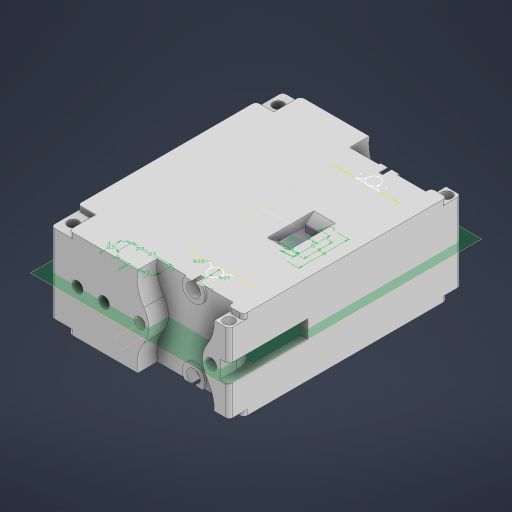
# Autodesk Inventor part: NEW_BODY
Saved by Autodesk Inventor 2024.2 (Build 282272000, 272)
## iProperties
Created: 2024-03-12
Part Number: NEW_BODY
Material: Generic
Document SubType Name: Modeling
Designer: jerem
Density: 1 g/cm^3
Appearance: Default
Author: jerem
## iProperties of the stored document NEW_BODY_3DPrint.ipt
Created: 2024-03-13
Part Number: NEW_BODY_3DPrint
Material: Generic
Document SubType Name: Modeling
Designer: jerem
Density: 1 g/cm^3
Appearance: Default
Author: jerem
Autodesk Inventor part; units mm, degrees
ref_plane "YZ Plane" through (0, 0, 0) normal (1, 0, 0) x (0, 1, 0)
ref_plane "XZ Plane" through (0, 0, 0) normal (0, 1, 0) x (-1, 0, 0)
ref_plane "XY Plane" through (0, 0, 0) normal (0, 0, 1) x (1, 0, 0)
sketch "Sketch1" plane through (0, 0, 0) normal (0, 1, 0) x (-1, 0, 0)
  line L0 (-50, -65) -> (50, -65)
  line L1 (50, -65) -> (50, 65)
  line L2 (50, 65) -> (-50, 65)
  line L3 (-50, 65) -> (-50, -65)
  line L4 (-50, -65) -> (50, 65) construction
  line L5 (50, -65) -> (-50, 65) construction
  point P0 (0, 0)
  dimension "d0" = 130
  dimension "d1" = 100
  constraints: 12 end point, 2 midpoint, 2 parallel, 1 horizontal, 1 perpendicular
  measures "d0" distance of L0.end L1.end
  measures "d1" distance of L1.end L2.end
extrude "Extrusion1" add sketch "Sketch1" along normal blind 50
sketch "Sketch2" plane through (-50, 0, 65) normal (0, 0, 1) x (1, 0, 0)
  line L0 (0, 50) -> (100, 50) projected
  line L1 (100, 50) -> (50, 50)
  line L2 (50, 50) -> (50, 0)
  line L3 (50, 0) -> (100, 0)
  line L4 (100, 0) -> (100, 50)
  constraints: 8 end point, 2 parallel, 1 horizontal, 1 perpendicular
extrude "Extrusion2" cut sketch "Sketch2" against normal blind 15
sketch "Sketch3" plane through (-50, 0, 50) normal (0, 0, 1) x (1, 0, 0)
  circle A0 centre (70, 46.3) radius 3.7
  line L0 (100, 50) -> (100, 0) projected
  line L1 (50, 50) -> (100, 50) projected
  line L2 (50, 0) -> (50, 50) projected
  line L3 (50, 25) -> (100, 25) construction
  circle A1 centre (70, 3.7) radius 3.7
  dimension "d8" = 7.4
  dimension "d95" = 20
  constraints: 2 centre point, 2 end point, 2 midpoint, 1 symmetric about line, 1 tangent, 1 other
  measures "d8" diameter of A0
  measures "d95" distance from line of L2 A0.centre
sketch "Sketch4" plane through (-50, 0, 50) normal (0, 0, 1) x (1, 0, 0)
  circle A0 centre (70, 46.3) radius 3.7 projected
  circle A1 centre (70, 3.7) radius 3.7 projected
  arc A2 (66.7875, 50) -> (73.2125, 50) centre (70, 46.3) ccw
  arc A3 (73.2125, 0) -> (66.7875, 0) centre (70, 3.7) ccw
  line L0 (73.2125, 50) -> (66.7875, 50)
  line L1 (50, 50) -> (100, 50) projected
  line L2 (73.2125, 0) -> (66.7875, 0)
  point P0 (50, 0)
  point P1 (70, 50)
  dimension "d11" = 1.2
  dimension "d12" = 1.2
  dimension "d13" = 6.4249
  dimension "d14" = 6.4249
  constraints: 4 end point, 4 point on circle, 2 centre point, 2 coincident, 1 parallel, 1 point on line, 1 vertical alignment
  measures "d12" radial gap between concentric circles of A1 A3
  measures "d13" distance of L0.start L0.end
  measures "d14" distance of L2.start L2.end
ref_plane "Work Plane1" through (50, 0, 0) normal (0, 0, -1) x (-1, 0, 0)
mirror "Mirror1" about plane through (50, 0, 0) normal (0, 0, -1) of "Extrusion2"
sketch "Sketch5" plane through (0, 0, 0) normal (0, -1, 0) x (1, 0, 0)
  line L0 (-46, -47.5) -> (-4, -47.5)
  line L1 (-4, -47.5) -> (-4, 47.5)
  line L2 (-4, 47.5) -> (-46, 47.5)
  line L3 (-46, 47.5) -> (-46, -47.5)
  line L4 (-46, -47.5) -> (-4, 47.5) construction
  line L5 (-4, -47.5) -> (-46, 47.5) construction
  line L6 (-50, -65) -> (-50, 65) projected
  line L7 (50, 50) -> (50, -50) projected
  line L8 (50, 0) -> (-50, 0) construction
  point P0 (0, 0)
  point P1 (-25, 0)
  dimension "d18" = 4
  dimension "d19" = 42
  dimension "d20" = 95
  constraints: 14 end point, 4 midpoint, 2 parallel, 1 horizontal, 1 perpendicular, 1 point on line
  measures "d18" distance between parallel lines of L6 L3
  measures "d19" distance of L1.end L2.end
  measures "d20" distance of L0.end L1.end
extrude "Extrusion5" cut sketch "Sketch5" against normal blind 30
sketch "Sketch6" plane through (0, 30, 0) normal (0, -1, 0) x (1, 0, 0)
  circle A0 centre (-7.75, -43.75) radius 1.7
  circle A1 centre (-42.25, -43.75) radius 1.7
  circle A2 centre (-42.25, 10.65) radius 1.7
  line L0 (-4, 47.5) -> (-4, -47.5) projected
  line L1 (-46, -47.5) -> (-46, 47.5) projected
  circle A3 centre (-42.25, 10.65) radius 3.75
  circle A4 centre (-42.25, -43.75) radius 3.75
  circle A5 centre (-7.75, -43.75) radius 3.75
  line L2 (-7.75, -43.75) -> (-4, -43.75)
  line L3 (-42.25, -43.75) -> (-46, -43.75)
  line L4 (-4, -47.5) -> (-46, -47.5) projected
  arc A6 (-14.4582, -47.5) -> (-11.4768, -44.1667) centre (-14.4582, -44.5) ccw
  arc A7 (-7.3333, -40.0232) -> (-4, -37.0418) centre (-7, -37.0418) ccw
  arc A8 (-46, -37.0418) -> (-42.6667, -40.0232) centre (-43, -37.0418) ccw
  arc A9 (-38.5232, -44.1667) -> (-35.5418, -47.5) centre (-35.5418, -44.5) ccw
  arc A10 (-42.6667, 6.9232) -> (-46, 3.9418) centre (-43, 3.9418) ccw
  arc A11 (-46, 17.3582) -> (-42.6667, 14.3768) centre (-43, 17.3582) ccw
  point P0 (0, 0)
  point P1 (-42.25, -47.5)
  point P2 (-7.75, -47.5)
  point P3 (-46, 10.65)
  dimension "d23" = 3.4
  dimension "d24" = 3.4
  dimension "d25" = 3.4
  dimension "d26" = 34.5
  dimension "d28" = 54.4
  dimension "d30" = 34.5
  dimension "d34" = 3
  dimension "d35" = 3
  dimension "d36" = 3
  dimension "d37" = 3
  dimension "d38" = 3
  dimension "d39" = 3
  constraints: 20 point on circle, 17 tangent, 12 centre point, 8 point on line, 4 end point, 3 coincident, 1 collinear
  measures "d23" diameter of A2
  measures "d24" diameter of A0
  measures "d25" diameter of A1
  measures "d26" distance of A1.centre A0.centre
  measures "d28" distance of A2.centre A1.centre
  measures "d30" horizontal distance of A0.centre A2.centre
  measures "d34" radius of A11
  measures "d35" radius of A10
  measures "d36" radius of A8
  measures "d37" radius of A9
  measures "d38" radius of A6
  measures "d39" radius of A7
extrude "Extrusion6" add sketch "Sketch6" along normal blind 8 from surface at 0
sketch "Sketch7" plane through (0, 50, 0) normal (0, 1, 0) x (1, 0, 0)
  line L0 (-46, 47.5) -> (-46, -47.5) projected
  line L1 (-46, -47.5) -> (-4, -47.5) projected
  line L2 (-4, -47.5) -> (-4, 47.5) projected
  line L3 (-4, 47.5) -> (-46, 47.5) projected
  line L4 (3, 41) -> (40, 41)
  line L5 (40, 41) -> (40, -41)
  line L6 (40, -41) -> (3, -41)
  line L7 (3, -41) -> (3, 41)
  line L8 (3, 41) -> (40, -41) construction
  line L9 (40, 41) -> (3, -41) construction
  line L10 (-46, 0) -> (-4, 0) construction
  line L11 (-4, -47.5) -> (-4, 47.5) construction
  line L12 (-50, 65) -> (-50, -65) projected
  line L13 (50, -50) -> (50, 50) projected
  point P0 (0, 0)
  point P1 (21.5, 0)
  point P2 (-4, 37.0418)
  dimension "d49" = 37
  dimension "d50" = 82
  dimension "d75" = 10
  constraints: 14 end point, 4 midpoint, 2 parallel, 2 perpendicular, 1 horizontal, 1 point on line
  measures "d49" distance of L5.end L6.end
  measures "d50" distance of L4.end L5.end
  measures "d75" distance between parallel lines of L13 L5
extrude "Extrusion7" cut sketch "Sketch7" against normal blind 30 contours L4 L5 L6 L7
sketch "Sketch9" plane through (0, 50, 0) normal (0, 1, 0) x (1, 0, 0)
  circle A0 centre (21.5, -44.5) radius 3.5
  line L0 (40, -41) -> (3, -41) projected
  line L1 (21.5, -44.5) -> (21.5, -41) construction
  line L2 (3, -41) -> (40, -41) construction
  arc A1 (28.5, -41) -> (25, -44.5) centre (28.5, -44.5) ccw
  arc A2 (18, -44.5) -> (14.5, -41) centre (14.5, -44.5) ccw
  line L3 (40, 41) -> (40, -41) construction
  line L4 (40, 0) -> (3, 0) construction
  line L5 (3, -41) -> (3, 41) construction
  circle A3 centre (21.5, 44.5) radius 3.5
  line L6 (21.5, 44.5) -> (21.5, 41) construction
  arc A4 (25, 44.5) -> (28.5, 41) centre (28.5, 44.5) ccw
  arc A5 (14.5, 41) -> (18, 44.5) centre (14.5, 44.5) ccw
  line L7 (28.5, 41) -> (14.5, 41)
  line L8 (3, 41) -> (40, 41) projected
  point P0 (0, 0)
  point P1 (14.5, -41)
  dimension "d60" = 7
  dimension "d62" = 3.5
  dimension "d63" = 3.5
  constraints: 14 point on circle, 10 end point, 9 symmetric about line, 6 centre point, 5 tangent, 4 midpoint, 4 point on line, 2 collinear, 3 other
  measures "d60" diameter of A0
  measures "d62" radius of A1
  measures "d63" radius of A2
sketch "Sketch10" plane through (0, 0, 0) normal (0, -1, 0) x (1, 0, 0)
  line L0 (-46, -47.5) -> (-46, 47.5) construction
  line L1 (-46, 0) -> (0, 0) construction
  line L2 (-4, -47.5) -> (-46, -47.5) projected
  line L3 (-46, -47.5) -> (-4, -47.5) construction
  circle A0 centre (-25, -52.5) radius 5
  arc A1 (-30, -52.5) -> (-35, -47.5) centre (-35, -52.5) ccw
  arc A2 (-15, -47.5) -> (-20, -52.5) centre (-15, -52.5) ccw
  line L4 (-25, -47.5) -> (-25, -52.5) construction
  line L5 (-4, -47.5) -> (-46, -47.5) construction
  line L6 (-4, 47.5) -> (-46, 47.5)
  line L7 (-46, 47.5) -> (-4, 47.5) construction
  circle A3 centre (-25, 52.5) radius 5
  arc A4 (-35, 47.5) -> (-30, 52.5) centre (-35, 52.5) ccw
  arc A5 (-20, 52.5) -> (-15, 47.5) centre (-15, 52.5) ccw
  line L8 (-25, 47.5) -> (-25, 52.5) construction
  line L9 (-14.4582, 47.5) -> (-35.5418, 47.5) construction
  point P0 (-14.4582, -47.5)
  point P1 (-35.5418, -47.5)
  dimension "d66" = 10
  dimension "d67" = 5
  dimension "d68" = 5
  constraints: 14 end point, 12 point on circle, 12 symmetric about line, 6 centre point, 6 point on line, 5 tangent, 2 horizontal, 2 midpoint, 1 perpendicular, 3 other
  measures "d66" diameter of A0
  measures "d67" radius of A2
  measures "d68" radius of A1
extrude "Extrusion10" cut sketch "Sketch10" against normal blind 3
sketch "Sketch11" plane through (0, 3, 0) normal (0, -1, 0) x (1, 0, 0)
  line L0 (-15, 47.5) -> (-35, 47.5) projected
  arc A0 (-20, 52.5) -> (-15, 47.5) centre (-15, 52.5) ccw projected
  arc A1 (-20, 52.5) -> (-30, 52.5) centre (-25, 52.5) ccw projected
  arc A2 (-35, 47.5) -> (-30, 52.5) centre (-35, 52.5) ccw projected
  line L1 (-35, -47.5) -> (-15, -47.5) projected
  arc A3 (-30, -52.5) -> (-35, -47.5) centre (-35, -52.5) ccw projected
  arc A4 (-30, -52.5) -> (-20, -52.5) centre (-25, -52.5) ccw projected
  arc A5 (-15, -47.5) -> (-20, -52.5) centre (-15, -52.5) ccw projected
  circle A6 centre (-25, -52.5) radius 1.5
  circle A7 centre (-25, 52.5) radius 1.5
  point P0 (0, 0)
  dimension "d71" = 3
  dimension "d72" = 3
  constraints: 2 centre point, 2 coincident
  measures "d71" diameter of A6
  measures "d72" diameter of A7
extrude "Extrusion11" cut sketch "Sketch11" against normal blind 5 contours A6 | A7
sketch "Sketch13" plane through (0, 20, 0) normal (0, 1, 0) x (1, 0, 0)
  line L0 (3, -41) -> (3, 41) projected
  line L1 (3, -41) -> (13, -41)
  line L2 (13, -41) -> (13, -21)
  line L3 (13, -21) -> (3, -21)
  line L4 (3, -21) -> (3, -41)
  point P0 (0, 0)
  point P1 (3, -21)
  dimension "d76" = 20
  dimension "d77" = 10
  constraints: 8 end point, 2 parallel, 1 horizontal, 1 perpendicular
  measures "d76" distance of L1.end L2.end
  measures "d77" distance of L2.end L3.end
revolve "Revolution1" cut sketch "Sketch13" angle 225 about axis through (3, 20, 41) along (0, 0, 1)
ref_plane "Work Plane5" through (0, 47, 0) normal (0, 1, 0) x (1, 0, 0)
sketch "Sketch16" plane through (40, 50, -41) normal (-1, 0, 0) x (0, 0, 1)
  line L0 (47.9232, -20) -> (48.917, -28) projected
  line L1 (0, -30) -> (82, -30) projected
  line L2 (82, -30) -> (62, -30)
  line L3 (62, -30) -> (62, -20)
  line L4 (62, -20) -> (82, -20)
  line L5 (82, -20) -> (82, -30)
  point P0 (41, -50)
  dimension "d83" = 20
  dimension "d84" = 10
  constraints: 8 end point, 2 parallel, 1 horizontal, 1 perpendicular
  measures "d83" distance of L3.end L4.end
  measures "d84" distance of L2.end L3.end
extrude "Extrusion13" cut sketch "Sketch16" against normal up to surface (10 mm away)
sketch "Sketch17" plane through (-50, 0, -65) normal (0, 0, -1) x (-1, 0, 0)
  line L0 (0, 0) -> (0, 50) construction
  line L1 (0, 25) -> (-15, 25) construction
  circle A0 centre (-15, 25) radius 3
  line L2 (-15, 25) -> (-29.8, 25) construction
  circle A1 centre (-29.8, 25) radius 3
  point P0 (-50, 0)
  dimension "d87" = 6
  dimension "d88" = 15
  dimension "d145" = 6
  dimension "d146" = 14.8
  constraints: 4 end point, 2 centre point, 2 coincident, 2 horizontal, 1 midpoint
  measures "d87" diameter of A0
  measures "d88" distance of L1.start L1.end
  measures "d145" diameter of A1
  measures "d146" distance of L2.start L2.end
extrude "Extrusion14" cut sketch "Sketch17" against normal blind 10
mirror "Mirror2" about plane through (0, 0, 0) normal (0, 0, 1) of "Extrusion14"
ref_plane "Work Plane3" through (16.7875, 0, -50) normal (0, 0, -1) x (-1, 0, 0)
sketch "Sketch18" plane through (16.7875, 0, -50) normal (0, 0, -1) x (-1, 0, 0)
  circle A0 centre (-3.2125, 46.3) radius 17.5 construction
  circle A1 centre (-3.2125, 3.7) radius 17.5 construction
  line L0 (-33.2125, 50) -> (-33.2125, 0) projected
  line L1 (-33.2125, 0) -> (-33.2125, 50)
  arc A2 (-33.2125, 10) -> (-33.2125, 40) centre (-33.2125, 25) ccw
  line L2 (26.8875, 50) -> (26.8875, 0)
  arc A3 (26.8875, 40) -> (26.8875, 10) centre (26.8875, 25) ccw
  point P0 (16.7875, 0)
  point P1 (-33.2125, 10)
  point P2 (26.8875, 10)
  point P3 (26.8875, 40)
  dimension "d91" = 35
  dimension "d92" = 35
  dimension "d96" = 30
  constraints: 4 centre point, 4 end point, 4 point on circle, 2 point on line, 1 midpoint
  measures "d91" diameter of A0
  measures "d92" diameter of A1
  measures "d96" diameter of A2
extrude "Extrusion15" add sketch "Sketch18" along normal up to surface (15 mm away)
ref_plane "Work Plane4" through (50, 25, -65) normal (0, 0, -1) x (-1, 0, 0)
sketch "Sketch19" plane through (50, 25, -65) normal (0, 0, -1) x (-1, 0, 0)
  arc A0 (0, -15) -> (0, 15) centre (0, 0) ccw construction
  line L0 (0, -15) -> (0, 15) construction
  circle A1 centre (10, 0) radius 3
  circle A2 centre (85, 0) radius 3 construction
  circle A3 centre (50.1, 0) radius 3
  line L1 (15, 0) -> (10, 0)
  arc A4 (50, 11.0901) -> (50, -11.0901) centre (60.1, 0) ccw projected
  line L2 (105.9, -25) -> (-17.65, -25) projected
  point P0 (45.1, 0)
  dimension "d97" = 6
  dimension "d101" = 6
  dimension "d102" = 5
  dimension "d144" = 5
  constraints: 2 centre point, 2 end point, 2 point on circle, 1 coincident, 1 midpoint, 1 parallel, 1 point on line
  measures "d97" diameter of A1
  measures "d101" diameter of A3
  measures "d102" distance of L1.start L1.end
  measures "d144" distance of point (45.1, 0) A3.centre
extrude "Extrusion16" cut sketch "Sketch19" against normal blind 10
sketch "Sketch21" plane through (0, 30, 0) normal (0, -1, 0) x (1, 0, 0)
  line L0 (-34, 47.5) -> (-16, 47.5)
  line L1 (-16, 47.5) -> (-16, 35.3)
  line L2 (-16, 35.3) -> (-34, 35.3)
  line L3 (-34, 35.3) -> (-34, 47.5)
  line L4 (-34, 47.5) -> (-46, 47.5) construction
  line L5 (-46, -47.5) -> (-46, 47.5) construction
  line L6 (-16, 47.5) -> (-4, 47.5) construction
  line L7 (-4, 47.5) -> (-4, -47.5) construction
  line L8 (-15, 47.5) -> (-35, 47.5) construction
  circle A0 centre (-36.25, 41.4) radius 1.5
  circle A1 centre (-13.75, 41.4) radius 1.5
  line L9 (-34, 41.4) -> (-36.25, 41.4)
  line L10 (-16, 41.4) -> (-13.75, 41.4)
  line L11 (-34, 47.5) -> (-38.75, 47.5)
  line L12 (-38.75, 47.5) -> (-38.75, 35.3)
  line L13 (-38.75, 35.3) -> (-11.25, 35.3)
  line L14 (-11.25, 35.3) -> (-11.25, 47.5)
  line L15 (-16, 47.5) -> (-11.25, 47.5)
  point P0 (0, 0)
  dimension "d108" = 18
  dimension "d110" = 0
  dimension "d202" = 3
  dimension "d203" = 22.5
  dimension "d206" = 3
  dimension "d207" = 12.2
  dimension "d208" = 27.5
  constraints: 26 end point, 6 point on line, 4 collinear, 4 perpendicular, 3 horizontal, 2 centre point, 2 midpoint, 2 parallel, 1 vertical
  measures "d108" distance of L0.start L0.end
  measures "d110" distance between parallel lines of L8 L0
  measures "d202" diameter of A0
  measures "d203" distance of L10.end L9.end
  measures "d206" diameter of A1
  measures "d207" distance of L11.end L12.end
  measures "d208" distance of L12.end L13.end
sketch "Sketch25" plane through (0, 50, 0) normal (0, 1, 0) x (1, 0, 0)
  line L0 (0, 65) -> (-50, 65) projected
  line L1 (-50, 65) -> (-40, 65)
  line L2 (-40, 65) -> (-40, 50)
  line L3 (-40, 50) -> (-50, 50)
  line L4 (-50, 50) -> (-50, 65)
  circle A0 centre (-45, 57.5) radius 3
  line L5 (-50, 65) -> (-50, -65) construction
  line L6 (-50, 0) -> (-20.5898, 0) construction
  point P0 (0, 0)
  point P1 (-30.8869, 65)
  dimension "d129" = 15
  dimension "d130" = 10
  dimension "d131" = 7.5
  dimension "d132" = 6
  dimension "d133" = 5
  constraints: 10 end point, 2 horizontal, 2 parallel, 1 centre point, 1 midpoint, 1 perpendicular
  measures "d129" distance of L1.end L2.end
  measures "d130" distance of L2.end L3.end
  measures "d131" distance from line of L3 A0.centre
  measures "d132" diameter of A0
  measures "d133" distance from line of L2 A0.centre
extrude "Extrusion21" cut sketch "Sketch25" against normal blind 3 contours L2 L3 L4 L0 | A0
extrude "Extrusion22" cut sketch "Sketch25" against normal blind 5 from surface at -3 contours A0
mirror "Mirror4" about plane through (0, 0, 0) normal (0, 0, 1) of "Extrusion21", "Extrusion22"
sketch "Sketch26" plane through (-10.1, 25, -65) normal (0, 0, -1) x (0, -1, 0)
  arc A0 (-11.0901, -10.1) -> (11.0901, -10.1) centre (0, 0) ccw projected
  circle A1 centre (0, -10) radius 3 projected
  circle A2 centre (0, -10) radius 3
  line L0 (0, -10) -> (-11.1803, -10) construction
  line L1 (0, -10) -> (11.1803, -10) construction
  line L2 (-22, 39.9) -> (-22, 29.9) projected
  line L3 (-22, 29.9) -> (-25, 29.9) projected
  line L4 (-25, -10.1) -> (-25, 29.9) projected
  line L5 (-25, -10.1) -> (-11.0901, -10.1) projected
  line L6 (11.0901, -10.1) -> (25, -10.1) projected
  line L7 (25, -10.1) -> (25, 39.9) projected
  line L8 (25, 39.9) -> (-22, 39.9) projected
  point P0 (-10.1, -25)
  constraints: 4 end point, 2 collinear, 2 point on circle, 1 centre point, 1 concentric, 1 horizontal, 1 point on line
extrude "Extrusion23" cut sketch "Sketch26" against normal up to surface (10 mm away) contours A1
ref_plane "Work Plane2" through (0, 25, 0) normal (0, -1, 0) x (1, 0, 0)
mirror "Mirror6" about plane through (0, 25, 0) normal (0, -1, 0) of "Extrusion21", "Extrusion22", "Mirror4"
sketch "Sketch27" plane through (-50, 47, -65) normal (-1, 0, 0) x (0, 0, 1)
  circle A0 centre (65, -22) radius 5
  line L0 (0, -44) -> (0, 0) projected
  line L1 (156, -22) -> (-26, -22) projected
  point P0 (65, -47)
  dimension "d140" = 10
  dimension "d141" = 65
  constraints: 1 centre point, 1 midpoint
  measures "d140" diameter of A0
  measures "d141" distance from line of L0 A0.centre
extrude "Extrusion24" cut sketch "Sketch27" against normal blind 5
mirror "Mirror7" about plane through (0, 0, 0) normal (0, 0, 1) of "Extrusion15"
sketch "Sketch28" plane through (50, 0, -50) normal (0, 0, -1) x (-1, 0, 0)
  circle A0 centre (10, 25) radius 3 projected
  line L0 (10, 25) -> (30, 25) construction
  line L1 (30, 25) -> (30, 46) construction
  circle A1 centre (30, 46) radius 3.5
  circle A2 centre (30, 46) radius 6.5
  line L2 (35.1235, 50) -> (24.8765, 50)
  line L3 (35.5, 50) -> (32, 50) projected
  line L4 (0, 50) -> (50, 50) projected
  line L5 (30, 49.5) -> (30, 50)
  line L6 (25, 50) -> (32, 50) projected
  line L7 (29, 50) -> (29, 49.3541)
  line L8 (31, 50) -> (31, 49.3541)
  point P0 (50, 0)
  dimension "d147" = 20
  dimension "d148" = 21
  dimension "d149" = 7
  dimension "d150" = 3
  dimension "d237" = 1
  constraints: 12 end point, 4 point on circle, 3 perpendicular, 3 point on line, 2 centre point, 2 coincident, 2 symmetric about line, 1 collinear, 1 horizontal, 1 line through centre
  measures "d147" distance of L0.start L0.end
  measures "d148" distance of L0.end L1.end
  measures "d149" diameter of A1
  measures "d150" radial gap between concentric circles of A2 A1
  measures "d237" distance between parallel lines of L5 L7
extrude "Extrusion25" add sketch "Sketch28" along normal blind 5 contours A1 L8 L2 A2 L7
mirror "Mirror8" about plane through (0, 25, 0) normal (0, -1, 0) of "Extrusion25"
mirror "Mirror9" about plane through (0, 0, 0) normal (0, 0, 1) of "Extrusion25", "Mirror8"
mirror "Mirror10" about plane through (0, 0, 0) normal (0, 0, 1) of "Extrusion16"
sketch "Sketch29" plane through (-10.1, 25, -65) normal (0, 0, -1) x (-1, 0, 0)
  arc A0 (-10.1, 11.0901) -> (-10.1, -11.0901) centre (0, 0) ccw projected
  line L0 (29.9, -25) -> (-10.1, -25) projected
  arc A1 (-8.7702, -25) -> (-12.3019, -8.5827) centre (-30.1, -21) ccw
  arc A2 (-29.1, -24.3541) -> (-31.1, -24.3541) centre (-30.1, -21) ccw projected
  constraints: 3 point on circle, 1 centre point, 1 concentric, 1 point on line, 1 tangent
sketch "Sketch31" plane through (-50, 0, 50) normal (0, 0, 1) x (1, 0, 0)
  line L0 (100, 50) -> (100, 40) projected
  arc A0 (100, 40) -> (100, 10) centre (100, 25) ccw projected
  line L1 (100, 50) -> (100, 40)
  line L2 (75.1235, 50) -> (100, 50) construction
  arc A1 (87.7115, 33.6019) -> (91.2464, 50) centre (70, 46) ccw
  line L3 (100, 50) -> (91.2464, 50)
  arc A2 (69, 49.3541) -> (71, 49.3541) centre (70, 46) ccw projected
  point P0 (50, 0)
  constraints: 4 end point, 3 point on circle, 1 centre point, 1 collinear, 1 concentric, 1 point on line, 1 tangent, 1 vertical
extrude "Extrusion28" add sketch "Sketch31" along normal up to surface (15 mm away)
mirror "Mirror13" about plane through (0, 25, 0) normal (0, -1, 0) of "Extrusion28"
mirror "Mirror14" about plane through (0, 0, 0) normal (0, 0, 1) of "Extrusion28", "Mirror13"
sketch "Sketch32" plane through (-10.1, 25, -65) normal (0, 0, -1) x (-1, 0, 0)
  arc A0 (-29.1, -24.3541) -> (-31.1, -24.3541) centre (-30.1, -21) ccw construction
  line L0 (-30.1, -21) -> (-30.1, 21.2793) construction
  line L1 (-35.1, 22) -> (-28.1, 22) construction
  arc A1 (-8.7702, -25) -> (-12.3019, -8.5827) centre (-30.1, -21) ccw
  arc A2 (-10.1, 11.0901) -> (-10.1, -11.0901) centre (0, 0) ccw projected
  line L2 (-10.1, -25) -> (-10.1, -11.0901)
  line L3 (-10.1, -11.0901) -> (-10.1, -25) construction
  line L4 (-24.9765, -25) -> (-10.1, -25) projected
  line L5 (-10.1, -25) -> (-8.7702, -25)
  point P0 (-51.3464, -25)
  point P1 (-10.1, -12.5762)
  constraints: 8 end point, 3 point on circle, 2 collinear, 1 centre point, 1 concentric, 1 perpendicular, 1 tangent
extrude "Extrusion29" add sketch "Sketch32" against normal up to surface (15 mm away) contours A1 A2 L2
extrude "Extrusion30" cut sketch "Sketch32" against normal up to surface (15 mm away) contours L5 L2 A1
mirror "Mirror15" about plane through (0, 25, 0) normal (0, -1, 0) of "Extrusion29", "Extrusion30"
mirror "Mirror16" about plane through (0, 0, 0) normal (0, 0, 1) of "Extrusion29", "Extrusion30", "Mirror15"
sketch "Sketch33" plane through (50, 0, -65) normal (1, 0, 0) x (0, 0, -1)
  line L0 (-106, 20) -> (-86, 20) projected
  line L1 (-130, 33.6019) -> (-130, 16.3981) projected
  line L2 (-106, 20) -> (-130, 20)
  line L3 (-130, 20) -> (-130, 30)
  line L4 (-130, 30) -> (-106, 30)
  line L5 (-106, 30) -> (-106, 20)
  point P0 (-65, 0)
  dimension "d167" = 10
  constraints: 8 end point, 2 parallel, 1 horizontal, 1 perpendicular, 1 point on line
  measures "d167" distance of L4.end L0.start
extrude "Extrusion31" cut sketch "Sketch33" against normal blind 5
sketch "Sketch34" plane through (0, 0, 0) normal (0, -1, 0) x (1, 0, 0)
  line L0 (50, 65) -> (50, -65) projected
  line L1 (50, -65) -> (41, -65)
  line L2 (41, -65) -> (41, -57)
  line L3 (41, -57) -> (50, -57)
  line L4 (50, -57) -> (50, -65)
  point P0 (0, 0)
  dimension "d170" = 9
  dimension "d171" = 8
  constraints: 8 end point, 2 parallel, 1 horizontal, 1 perpendicular
  measures "d170" distance of L0.end L1.end
  measures "d171" distance of L1.end L2.end
extrude "Extrusion32" cut sketch "Sketch34" against normal blind 3
sketch "Sketch35" plane through (0, 3, 0) normal (0, -1, 0) x (1, 0, 0)
  circle A0 centre (46, -61) radius 3
  line L0 (50, -57) -> (50, -65) projected
  line L1 (50, -65) -> (41.5965, -65) projected
  point P0 (0, 0)
  point P1 (42, -65)
  dimension "d174" = 6
  dimension "d175" = 4
  dimension "d176" = 4
  constraints: 1 centre point
  measures "d174" diameter of A0
  measures "d175" distance from line of L0 A0.centre
  measures "d176" distance from line of L1 A0.centre
extrude "Extrusion33" cut sketch "Sketch35" against normal blind 11
mirror "Mirror17" about plane through (0, 25, 0) normal (0, -1, 0) of "Extrusion32", "Extrusion33"
mirror "Mirror18" about plane through (0, 0, 0) normal (0, 0, 1) of "Extrusion32", "Extrusion33", "Mirror17"
sketch "Sketch37" plane through (40, 50, -41) normal (-1, 0, 0) x (0, 0, 1)
  line L0 (62, -30) -> (62, -20) projected
  line L1 (62, -20) -> (82, -20) projected
  line L2 (82, 0) -> (82, -20) projected
  line L3 (0, 0) -> (82, 0) projected
  line L4 (0, 0) -> (0, -30) projected
  line L5 (0, -30) -> (62, -30) projected
  line L6 (82, 0) -> (82, -20) projected
  line L7 (82, -5) -> (0, -5)
  point P0 (41, -50)
  point P1 (82, -5)
  dimension "d186" = 5
  constraints: 2 end point, 2 point on line, 1 perpendicular
  measures "d186" distance between parallel lines of L3 L7
extrude "Extrusion34" cut sketch "Sketch37" against normal blind 5 contours L5 L4 L7 L2 L1 L0
fillet "Fillet5" radius 15 1 edges at (45, 25, 41)
fillet "Fillet6" radius 2 17 edges at (50, 25, -65) (50, 11.5, 65) (50, 38.5, 65) (-50, 25, 65) (-50, 25, -65) (-40, 1.5, -65) (-50, 1.5, -50) (-50, 1.5, 50) (-40, 1.5, 65) (41.4739, 1.4939, 57) (41.4739, 48.5061, 57) (-40, 48.5, 65) (-50, 48.5, 50) (41.4739, 48.5061, -57) (-50, 48.5, -50) (-40, 48.5, -65) (41.4739, 1.4939, -57)
fillet "Fillet8" radius 2 4 edges at (50, 48.5, -57) (50, 1.5, -57) (50, 1.5, 57) (50, 48.5, 57)
sketch "Sketch39" plane through (0, 0, 0) normal (0, -1, 0) x (1, 0, 0)
  line L0 (-4, 47.5) -> (-4, -37.0418) projected
  circle A0 centre (-4, 0) radius 7
  point P0 (0, 0)
  point P1 (-4, 21)
  point P2 (-4, 7)
  point P3 (-4, -7)
  dimension "d192" = 14
  constraints: 1 centre point, 1 point on line
  measures "d192" diameter of A0
extrude "Extrusion36" cut sketch "Sketch39" against normal blind 3 contours A0 L0 picked at (-0.6441, -1.6274)
sketch "Sketch40" plane through (20, 46, 55) normal (0, 0, 1) x (1, 0, 0)
  arc A0 (-1, 3.3541) -> (1, 3.3541) centre (0, 0) ccw projected
  circle A1 centre (0, 0) radius 3.85
  point P0 (-20, -46)
  constraints: 1 centre point, 1 coincident
extrude "Extrusion37" cut sketch "Sketch40" against normal up to surface (5 mm away)
mirror "Mirror19" about plane through (0, 25, 0) normal (0, -1, 0) of "Extrusion37"
mirror "Mirror20" about plane through (0, 0, 0) normal (0, 0, 1) of "Extrusion37", "Mirror19"
sketch "Sketch42" plane through (0, 30, 0) normal (0, -1, 0) x (1, 0, 0)
  point P0 (0, 0)
sketch "Sketch43" plane through (0, 30, 0) normal (0, -1, 0) x (1, 0, 0)
  line L0 (-35, -47.5) -> (-15, -47.5)
  line L1 (-15, -47.5) -> (-15, 2.5)
  line L2 (-15, 2.5) -> (-35, 2.5)
  line L3 (-35, 2.5) -> (-35, -47.5)
  line L4 (-35, -47.5) -> (-15, 2.5) construction
  line L5 (-15, -47.5) -> (-35, 2.5) construction
  line L6 (-25, -22.5) -> (-4, -22.5) construction
  line L7 (-4, -7) -> (-4, -47.5) construction
  line L8 (-25, -22.5) -> (-46, -22.5) construction
  line L9 (-46, -47.5) -> (-46, 47.5) construction
  line L10 (-4, -47.5) -> (-15, -47.5) construction
  point P0 (0, 0)
  dimension "d222" = 50
  dimension "d223" = 20
  dimension "d224" = 0
  constraints: 16 end point, 3 point on line, 2 horizontal, 2 midpoint, 2 parallel, 1 collinear, 1 perpendicular
  measures "d222" distance of L0.end L1.end
  measures "d223" distance of L1.end L2.end
  measures "d224" distance between parallel lines of L10 L0
extrude "Extrusion42" cut sketch "Sketch43" against normal blind 7
sketch "Sketch44" plane through (0, 20, 0) normal (0, 1, 0) x (1, 0, 0)
  line L0 (3, -41) -> (-4, -41) projected
  line L1 (45, 41) -> (3, 41)
  line L2 (3, 41) -> (3, -41)
  line L3 (3, -41) -> (45, -41)
  line L4 (45, -41) -> (45, 41)
  point P0 (0, 0)
  constraints: 8 end point, 2 parallel, 1 horizontal, 1 perpendicular
extrude "Extrusion43" add sketch "Sketch44" along normal up to surface (30 mm away)
sketch "Sketch46" plane through (0, 30, 0) normal (0, -1, 0) x (1, 0, 0)
  line L0 (-15, 2.5) -> (-15, -47.5) projected
  line L1 (-14.4582, -47.5) -> (-15, -47.5) projected
  arc A0 (-14.4582, -47.5) -> (-11.4768, -44.1667) centre (-14.4582, -44.5) ccw projected
  arc A1 (-7.3333, -40.0232) -> (-4, -37.0418) centre (-7, -37.0418) ccw projected
  line L2 (-4, 47.5) -> (-4, -37.0418) projected
  line L3 (-46, 47.5) -> (-4, 47.5) projected
  line L4 (-46, 17.3582) -> (-46, 47.5) projected
  arc A2 (-46, 17.3582) -> (-42.6667, 14.3768) centre (-43, 17.3582) ccw projected
  arc A3 (-42.6667, 6.9232) -> (-46, 3.9418) centre (-43, 3.9418) ccw projected
  line L5 (-46, 0) -> (-46, 3.9418) projected
  line L6 (-46, -37.0418) -> (-46, 0) projected
  arc A4 (-46, -37.0418) -> (-42.6667, -40.0232) centre (-43, -37.0418) ccw projected
  arc A5 (-38.5232, -44.1667) -> (-35.5418, -47.5) centre (-35.5418, -44.5) ccw projected
  line L7 (-35, -47.5) -> (-35.5418, -47.5) projected
  line L8 (-35, -47.5) -> (-35, 2.5) projected
  line L9 (-35, 2.5) -> (-15, 2.5) projected
  line L10 (-46, 4) -> (-46, -5) projected
  line L11 (-46, -5) -> (-35, -5)
  line L12 (-42.6667, 14.3768) -> (-32.6667, 14.3768)
  line L13 (-32.6667, 14.3768) -> (-32.6667, 2.5)
  arc A6 (-7.3333, -40.0232) -> (-11.4768, -44.1667) centre (-7.75, -43.75) ccw projected
  arc A7 (-42.6667, 6.9232) -> (-42.6667, 14.3768) centre (-42.25, 10.65) ccw projected
  arc A8 (-38.5232, -44.1667) -> (-42.6667, -40.0232) centre (-42.25, -43.75) ccw projected
  line L14 (-42.6667, 14.3768) -> (-42.6667, 11.2818)
  point P0 (0, 0)
  point P1 (-46, -4.5826)
  point P2 (-46, 4.9552)
  point P3 (-46, -5)
  point P4 (-41.8333, 14.3768)
  dimension "d231" = 10
  constraints: 8 end point, 2 perpendicular, 2 point on line, 1 horizontal, 1 vertical
  measures "d231" distance of L12.start L12.end
extrude "Extrusion45" cut sketch "Sketch46" against normal up to surface (7 mm away)
sketch "Sketch47" plane through (0, 37, 0) normal (0, -1, 0) x (1, 0, 0)
  line L0 (-35.5418, -47.5) -> (-14.4582, -47.5) projected
  arc A0 (-14.4582, -47.5) -> (-11.4768, -44.1667) centre (-14.4582, -44.5) ccw projected
  arc A1 (-7.3333, -40.0232) -> (-11.4768, -44.1667) centre (-7.75, -43.75) ccw projected
  arc A2 (-7.3333, -40.0232) -> (-4, -37.0418) centre (-7, -37.0418) ccw projected
  line L1 (-4, -37.0418) -> (-4, 47.5) projected
  line L2 (-4, 47.5) -> (-46, 47.5) projected
  line L3 (-46, 47.5) -> (-46, 17.3582) projected
  arc A3 (-46, 17.3582) -> (-42.6667, 14.3768) centre (-43, 17.3582) ccw projected
  line L4 (-42.6667, 14.3768) -> (-41.8333, 14.3768) projected
  arc A4 (-42.6667, 6.9232) -> (-41.8333, 14.3768) centre (-42.25, 10.65) ccw projected
  arc A5 (-42.6667, 6.9232) -> (-46, 3.9418) centre (-43, 3.9418) ccw projected
  line L5 (-46, 3.9418) -> (-46, -37.0418) projected
  arc A6 (-46, -37.0418) -> (-42.6667, -40.0232) centre (-43, -37.0418) ccw projected
  arc A7 (-38.5232, -44.1667) -> (-42.6667, -40.0232) centre (-42.25, -43.75) ccw projected
  arc A8 (-38.5232, -44.1667) -> (-35.5418, -47.5) centre (-35.5418, -44.5) ccw projected
  point P0 (0, 0)
extrude "Extrusion46" cut sketch "Sketch47" against normal blind 2
sketch "Sketch51" plane through (-50, 0, 50) normal (0, 0, 1) x (1, 0, 0)
  arc A0 (48.6702, 50) -> (52.2019, 33.5827) centre (70, 46) ccw projected
  arc A1 (52.2019, 16.4173) -> (52.2019, 33.5827) centre (39.9, 25) ccw projected
  arc A2 (52.2019, 16.4173) -> (48.6702, 0) centre (70, 4) ccw projected
  line L0 (64.8765, 0) -> (48.6702, 0) projected
  arc A3 (75.1235, 0) -> (64.8765, 0) centre (70, 4) ccw projected
  line L1 (91.2464, 0) -> (75.1235, 0) projected
  arc A4 (91.2464, 0) -> (87.7115, 16.3981) centre (70, 4) ccw projected
  arc A5 (87.7115, 33.6019) -> (87.7115, 16.3981) centre (100, 25) ccw projected
  arc A6 (87.7115, 33.6019) -> (91.2464, 50) centre (70, 46) ccw projected
  line L2 (75.1235, 50) -> (91.2464, 50) projected
  arc A7 (64.8765, 50) -> (75.1235, 50) centre (70, 46) ccw projected
  line L3 (48.6702, 50) -> (64.8765, 50) projected
  point P0 (50, 0)
extrude "Extrusion47" add sketch "Sketch51" along normal blind 4
sketch "Sketch52" plane through (20, 46, -50) normal (0, 0, -1) x (-1, 0, 0)
  arc A0 (17.7981, -12.4173) -> (21.3298, 4) centre (0, 0) ccw projected
  line L0 (5.1235, 4) -> (21.3298, 4) projected
  arc A1 (-5.1235, 4) -> (5.1235, 4) centre (0, 0) ccw projected
  line L1 (-21.2464, 4) -> (-5.1235, 4) projected
  arc A2 (-21.2464, 4) -> (-17.7115, -12.3981) centre (0, 0) ccw projected
  arc A3 (-17.7115, -29.6019) -> (-17.7115, -12.3981) centre (-30, -21) ccw projected
  arc A4 (-17.7115, -29.6019) -> (-21.2464, -46) centre (0, -42) ccw projected
  line L2 (-5.1235, -46) -> (-21.2464, -46) projected
  arc A5 (5.1235, -46) -> (-5.1235, -46) centre (0, -42) ccw projected
  line L3 (21.3298, -46) -> (5.1235, -46) projected
  arc A6 (21.3298, -46) -> (17.7981, -29.5827) centre (0, -42) ccw projected
  arc A7 (17.7981, -12.4173) -> (17.7981, -29.5827) centre (30.1, -21) ccw projected
  point P0 (20, -46)
extrude "Extrusion48" add sketch "Sketch52" along normal blind 4
sketch "Sketch53" plane through (0, 0, 0) normal (0, -1, 0) x (1, 0, 0)
  line L0 (-46, -47.5) -> (-46, 47.5) projected
  line L1 (-46, 47.5) -> (46, 47.5)
  line L2 (46, 47.5) -> (46, -47.5)
  line L3 (46, -47.5) -> (-46, -47.5)
  line L4 (-46, -47.5) -> (-46, 47.5)
  line L5 (50, 55) -> (50, -55) projected
  point P0 (0, 0)
  dimension "d244" = 4
  constraints: 8 end point, 2 parallel, 1 horizontal, 1 perpendicular
  measures "d244" distance between parallel lines of L5 L2
extrude "Extrusion49" cut sketch "Sketch53" against normal blind 45
sketch "Sketch54" plane through (-46, 0, -47.5) normal (0, 0, 1) x (1, 0, 0)
  circle A0 centre (57.036, 7.7) radius 1.5
  line L0 (92, 5) -> (0, 5)
  line L1 (0, 5) -> (0, 45)
  line L2 (0, 45) -> (92, 45)
  line L3 (92, 45) -> (92, 5)
  line L4 (96, 47) -> (96, 3) projected
  line L5 (-4, 3) -> (-4, 47) projected
  line L6 (60.8765, 0) -> (44.6702, 0) projected
  line L7 (44.6702, 50) -> (8, 50) projected
  line L8 (59.736, 5) -> (59.736, 46.19) construction
  line L9 (-0.264, 5) -> (-0.264, 45) construction
  circle A1 centre (2.436, 7.7) radius 1.5
  line L10 (54.336, 10.4) -> (59.736, 10.4)
  line L11 (59.736, 10.4) -> (59.736, 5)
  line L12 (59.736, 5) -> (54.336, 5)
  line L13 (54.336, 5) -> (54.336, 10.4)
  line L14 (54.336, 10.4) -> (59.736, 5) construction
  line L15 (59.736, 10.4) -> (54.336, 5) construction
  line L16 (5.136, 10.4) -> (-0.264, 10.4)
  line L17 (-0.264, 10.4) -> (-0.264, 5)
  line L18 (-0.264, 5) -> (5.136, 5)
  line L19 (5.136, 5) -> (5.136, 10.4)
  line L20 (5.136, 10.4) -> (-0.264, 5) construction
  line L21 (-0.264, 10.4) -> (5.136, 5) construction
  line L22 (-0.264, 45) -> (5.136, 45) construction
  line L23 (5.136, 45) -> (5.136, 39.6)
  line L24 (5.136, 39.6) -> (-0.264, 39.6)
  line L25 (-0.264, 39.6) -> (-0.264, 45)
  circle A2 centre (2.436, 42.3) radius 1.5
  line L26 (2.436, 42.3) -> (2.436, 39.6) construction
  line L27 (2.436, 42.3) -> (5.136, 42.3) construction
  line L28 (59.736, 45) -> (54.336, 45) construction
  line L29 (54.336, 45) -> (54.336, 39.6)
  line L30 (54.336, 39.6) -> (59.736, 39.6)
  line L31 (59.736, 39.6) -> (59.736, 45)
  circle A3 centre (57.036, 42.3) radius 1.5
  point P0 (46, 0)
  point P1 (5.136, 5)
  point P2 (54.336, 5)
  point P3 (0, 10.4)
  point P4 (0, 5)
  point P5 (0, 39.6)
  point P6 (5.136, 45)
  dimension "d247" = 4
  dimension "d248" = 4
  dimension "d249" = 5
  dimension "d250" = 5
  dimension "d251" = 2.7
  dimension "d252" = 3
  dimension "d253" = 2.7
  dimension "d254" = 2.7
  dimension "d255" = 2.7
  dimension "d256" = 3
  dimension "d257" = 60
  dimension "d305" = 5.4
  dimension "d306" = 5.4
  dimension "d307" = 3
  dimension "d308" = 2.7
  dimension "d309" = 2.7
  dimension "d310" = 40
  dimension "d311" = 3
  constraints: 56 end point, 10 parallel, 7 perpendicular, 6 midpoint, 6 point on line, 5 horizontal, 4 centre point
  measures "d247" distance between parallel lines of L4 L3
  measures "d248" distance between parallel lines of L5 L1
  measures "d249" distance between parallel lines of L6 L0
  measures "d250" distance between parallel lines of L7 L2
  measures "d251" distance from line of L0 A0.centre
  measures "d252" diameter of A0
  measures "d253" distance from line of L8 A0.centre
  measures "d254" distance from line of L0 A1.centre
  measures "d255" distance from line of L9 A1.centre
  measures "d256" diameter of A1
  measures "d257" distance between parallel lines of L9 L8
  measures "d305" distance of L22.end L23.end
  measures "d306" distance of L23.end L24.end
  measures "d307" diameter of A2
  measures "d308" distance of L26.start L26.end
  measures "d309" distance of L26.start L27.end
  measures "d310" distance between parallel lines of L22 L0
  measures "d311" diameter of A3
extrude "Extrusion50" add sketch "Sketch54" against normal blind 14 from surface at 95 contours L0 L13 L10 L11 | L31 L30 L29 L2 | L23 L24 L1 L2
sketch "Sketch55" plane through (0, 45, 0) normal (0, -1, 0) x (1, 0, 0)
  line L0 (-46, 47.5) -> (46, 47.5) projected
  line L1 (-35, -47.5) -> (-46, -47.5) projected
  line L2 (-46, -47.5) -> (-46, -22.5)
  line L3 (-46, -47.5) -> (-46, 47.5) projected
  line L4 (-46, -22.5) -> (44, -22.5)
  line L5 (44, -22.5) -> (44, -47.5)
  line L6 (46, -47.5) -> (-46, -47.5) projected
  line L7 (46, -47.5) -> (46, -20.5)
  line L8 (46, -20.5) -> (-48, -20.5)
  line L9 (-48, -20.5) -> (-48, -47.5)
  line L10 (44, -22.5) -> (46, -22.5)
  point P0 (0, 0)
  point P1 (-46, -20.5)
  point P2 (46, -47.5)
  dimension "d262" = 25
  dimension "d263" = 90
  dimension "d264" = 2
  constraints: 14 end point, 5 perpendicular, 3 point on line, 2 other
  measures "d262" distance of L1.end L2.end
  measures "d263" distance of L2.end L4.end
  measures "d264" distance between parallel lines of L4 L8
extrude "Extrusion51" add sketch "Sketch55" along normal blind 43 contours L3 L8 L7 L10 L4
sketch "Sketch56" plane through (-46, 45, -20.5) normal (0, 0, 1) x (1, 0, 0)
  line L0 (90, -43) -> (80, -43)
  line L1 (80, -43) -> (80, -28)
  line L2 (80, -28) -> (90, -28)
  line L3 (90, -28) -> (90, -43)
  line L4 (92, -43) -> (0, -43) projected
  line L5 (92, 0) -> (92, -43) projected
  point P0 (46, -45)
  dimension "d268" = 15
  dimension "d269" = 10
  dimension "d312" = 0
  dimension "d313" = 2
  constraints: 8 end point, 2 parallel, 1 horizontal, 1 perpendicular
  measures "d268" distance of L2.end L0.start
  measures "d269" distance of L1.end L2.end
  measures "d312" distance between parallel lines of L4 L0
  measures "d313" distance between parallel lines of L5 L3
extrude "Extrusion52" cut sketch "Sketch56" against normal up to surface (2 mm away)
sketch "Sketch57" plane through (-50, 0, -48) normal (-1, 0, 0) x (0, 0, 1)
  line L0 (38, 30) -> (58, 30)
  line L1 (58, 30) -> (58, 20)
  line L2 (58, 20) -> (38, 20)
  line L3 (38, 20) -> (38, 30)
  circle A0 centre (48, 25) radius 5 projected
  line L4 (38, 30) -> (58, 20) construction
  line L5 (58, 30) -> (38, 20) construction
  point P0 (48, 0)
  dimension "d272" = 20
  dimension "d273" = 10
  constraints: 12 end point, 2 midpoint, 2 parallel, 1 horizontal, 1 perpendicular
  measures "d272" distance of L1.end L2.end
  measures "d273" distance of L0.end L1.end
extrude "Extrusion53" cut sketch "Sketch57" against normal up to surface (4 mm away)
sketch "Sketch58" plane through (0, 45, 0) normal (0, -1, 0) x (1, 0, 0)
  line L0 (19.3804, -14.1222) -> (31.3804, -14.1222)
  line L1 (31.3804, -14.1222) -> (31.3804, 13.8778)
  line L2 (31.3804, 13.8778) -> (19.3804, 13.8778)
  line L3 (19.3804, 13.8778) -> (19.3804, -14.1222)
  line L4 (19.3804, -14.1222) -> (31.3804, 13.8778) construction
  line L5 (31.3804, -14.1222) -> (19.3804, 13.8778) construction
  circle A0 centre (25.3804, 10.3778) radius 1.5
  circle A1 centre (25.3804, -10.6222) radius 1.5
  line L6 (25.3804, 10.3778) -> (25.3804, -0.1222) construction
  line L7 (25.3804, -10.6222) -> (25.3804, -0.1222) construction
  line L8 (19.3804, -8.1222) -> (31.3804, -8.1222)
  line L9 (31.3804, -8.1222) -> (31.3804, 7.8778)
  line L10 (31.3804, 7.8778) -> (19.3804, 7.8778)
  line L11 (19.3804, 7.8778) -> (19.3804, -8.1222)
  line L12 (19.3804, -8.1222) -> (31.3804, 7.8778) construction
  line L13 (31.3804, -8.1222) -> (19.3804, 7.8778) construction
  point P0 (0, 0)
  point P1 (25.3804, -14.1222)
  dimension "d276" = 3
  dimension "d278" = 21
  dimension "d279" = 3
  dimension "d280" = 12
  dimension "d281" = 6
  dimension "d282" = 6
  dimension "d283" = 28
  dimension "d284" = 16
  constraints: 28 end point, 4 midpoint, 4 parallel, 2 centre point, 2 horizontal, 2 perpendicular, 1 collinear, 1 point on line
  measures "d276" diameter of A0
  measures "d278" distance of L7.start L6.start
  measures "d279" diameter of A1
  measures "d280" distance between parallel lines of L3 L1
  measures "d281" distance from line of L1 L6.start
  measures "d282" distance from line of L1 L7.start
  measures "d283" distance between parallel lines of L0 L2
  measures "d284" distance between parallel lines of L8 L10
extrude "Extrusion54" add sketch "Sketch58" along normal blind 3 contours L3 L8 L1 L0 | L3 L2 L1 L10
extrude "Extrusion55" cut sketch "Sketch58" against normal up to surface (5 mm away) contours L3 L10 L1 L8
sketch "Sketch59" plane through (46, 0, -47.5) normal (-1, 0, 0) x (0, 0, 1)
  line L0 (47.5, 0) -> (42.5, 0)
  line L1 (95, 0) -> (0, 0) projected
  line L2 (42.5, 0) -> (42.5, 5)
  line L3 (42.5, 5) -> (52.5, 5)
  line L4 (52.5, 5) -> (52.5, 0)
  line L5 (52.5, 0) -> (47.5, 0)
  dimension "d289" = 5
  dimension "d290" = 5
  dimension "d291" = 10
  constraints: 10 end point, 2 perpendicular, 2 point on line, 1 collinear, 1 vertical
  measures "d289" distance of L0.start L0.end
  measures "d290" distance of L0.end L2.end
  measures "d291" distance of L2.end L3.end
extrude "Extrusion56" add sketch "Sketch59" along normal blind 10
sketch "Sketch60" plane through (0, 0, 0) normal (0, -1, 0) x (1, 0, 0)
  line L0 (46, 5) -> (36, 5) projected
  line L1 (46, -5) -> (36, -5) projected
  line L2 (36, 5) -> (46, 5)
  line L3 (46, 5) -> (46, -5)
  line L4 (46, -5) -> (36, -5)
  line L5 (36, -5) -> (36, 5)
  point P0 (0, 0)
  constraints: 8 end point, 2 parallel, 1 horizontal, 1 perpendicular
extrude "Extrusion57" cut sketch "Sketch60" against normal blind 2
sketch "Sketch61" plane through (0, 2, 0) normal (0, -1, 0) x (1, 0, 0)
  circle A0 centre (41, 0) radius 1.5
  point P0 (0, 0)
  dimension "d296" = 3
  constraints: 1 centre point
  measures "d296" diameter of A0
extrude "Extrusion58" cut sketch "Sketch61" against normal blind 3
chamfer "Chamfer6" distance 5 distance2 4 2 edges at (25.3804, 50, 7.8778) (25.3804, 50, -8.1222) measured on face at (25.3804, 50, 8.3778) measured on face at (25.3804, 50, -8.6222)
chamfer "Chamfer7" distance 6 distance2 6 1 edges at (46, 5, 0) measured on face at (46, 5.5, 0)
equation "\"d12\" = d11"
equation "\"d24\" = d23"
equation "\"d25\" = d23"
equation "\"d30\" = d26"
equation "\"d35\" = d34"
equation "\"d36\" = d34"
equation "\"d37\" = d34"
equation "\"d38\" = d34"
equation "\"d39\" = d34"
equation "\"d62\" = 0.5 * d60"
equation "\"d63\" = d62"
equation "\"d72\" = d71"
equation "\"M4_HOLE_D\" = 3.81"
equation "\"TOL\" = 0.04"
equation "\"M4_INSRT_D\" = 6"
body "Solid1"
